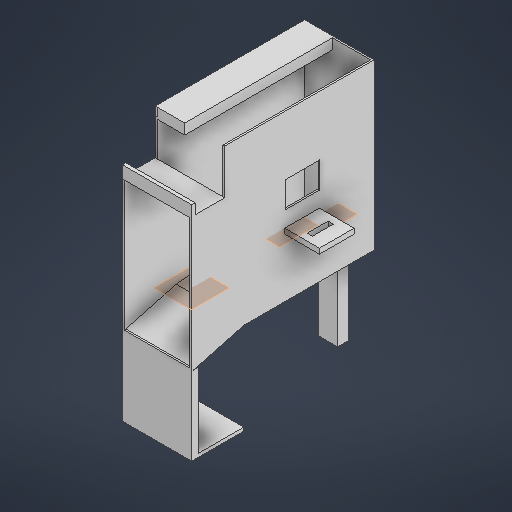
# Autodesk Inventor part: Na servo
Saved by Autodesk Inventor 2026.2 (Build 302298000, 298)
## iProperties
Created: 2026-03-13
Part Number: Na servo
Material: Všeobecné
Document SubType Name: Modeling
Designer: cerna
Density: 1 g/cm^3
Appearance: Výchozí
Author: cerna
Autodesk Inventor part; units mm, degrees
ref_plane "YZ Plane" through (0, 0, 0) normal (1, 0, 0) x (0, 1, 0)
ref_plane "XZ Plane" through (0, 0, 0) normal (0, 1, 0) x (-1, 0, 0)
ref_plane "XY Plane" through (0, 0, 0) normal (0, 0, 1) x (1, 0, 0)
sketch "Náčrt1" plane through (0, 0, 0) normal (0, 1, 0) x (-1, 0, 0)
  line L0 (20, 15) -> (-20, 15)
  line L1 (-20, 15) -> (-20, -15)
  line L2 (-20, -15) -> (20, -15)
  line L3 (20, -15) -> (20, 15)
  line L4 (0, -21) -> (0, 21) projected
  line L5 (-28, 0) -> (28, 0) projected
  point P0 (0, 0)
  dimension "d0" = 40
  dimension "d1" = 30
  constraints: 8 end point, 2 parallel, 1 horizontal, 1 perpendicular, 2 other
  measures "d0" distance of L2.end L1.end
  measures "d1" distance of L1.end L0.end
extrude "Vysunutí1" add sketch "Náčrt1" along normal blind 2
sketch "Náčrt2" plane through (0, 2, 0) normal (0, 1, 0) x (1, 0, 0)
  line L0 (-20, 15) -> (-20, -15) projected
  line L1 (-20, -15) -> (20, -15)
  line L2 (20, -15) -> (20, -14)
  line L3 (20, -14) -> (-20, -14)
  line L4 (-20, -14) -> (-20, -15)
  point P0 (0, 0)
  point P1 (-20, -14)
  dimension "d4" = 40
  dimension "d5" = 1
  constraints: 8 end point, 2 parallel, 1 horizontal, 1 perpendicular
  measures "d4" distance of L3.end L2.end
  measures "d5" distance of L2.end L1.end
extrude "Vysunutí2" add sketch "Náčrt2" along normal blind 44
sketch "Náčrt3" plane through (20, 0, 15) normal (1, 0, 0) x (0, 0, -1)
  line L0 (1, 2) -> (1, 46) projected
  line L1 (1, 45) -> (30.1328, 52.8061)
  line L2 (30.1328, 53.8061) -> (1, 46)
  line L3 (1, 46) -> (1, 45)
  line L4 (30.1328, 53.8061) -> (30.1328, 52.8061)
  line L5 (30, 0) -> (30, 2) projected
  line L6 (30.1328, 53.8061) -> (30.1328, 52.8061)
  line L7 (30.1328, 52.8061) -> (105.1328, 52.8061)
  line L8 (105.1328, 52.8061) -> (105.1328, 60.8061)
  line L9 (105.1328, 60.8061) -> (30.1328, 53.8061)
  point P0 (15, 0)
  point P1 (30.1328, 53.3061)
  dimension "d8" = 1
  dimension "d10" = 105
  dimension "d11" = 29.1328
  dimension "d59" = 75
  dimension "d60" = 8
  constraints: 16 end point, 2 perpendicular, 2 vertical, 1 collinear, 1 midpoint, 1 point on line
  measures "d8" distance of L1.start L0.end
  measures "d10" angle of L1 L0
  measures "d11" horizontal distance of L1.start L1.end
  measures "d59" distance of L1.end L7.end
  measures "d60" distance of L7.end L8.end
extrude "Vysunutí3" add sketch "Náčrt3" against normal blind 40
sketch "Náčrt5" plane through (20, 0, 15) normal (1, 0, 0) x (0, 0, -1)
  line L0 (53.6328, 89.524) -> (73.6328, 89.524)
  line L1 (73.6328, 89.524) -> (73.6328, 86.524)
  line L2 (73.6328, 86.524) -> (53.6328, 86.524)
  line L3 (53.6328, 86.524) -> (53.6328, 89.524)
  line L4 (0, 0) -> (30, 0) projected
  line L5 (30, 0) -> (30, 2) projected
  line L6 (1, 2) -> (30, 2) projected
  line L7 (1, 2) -> (1, 45) projected
  line L8 (1, 45) -> (30.1328, 52.8061) projected
  line L9 (30.1328, 53.8061) -> (1, 46) projected
  line L10 (0, 46) -> (1, 46) projected
  line L11 (0, 0) -> (0, 46) projected
  line L12 (67.1328, 89.524) -> (60.1328, 89.524) projected
  line L13 (63.6328, 89.524) -> (63.6328, 67.9806)
  line L14 (30.1328, 52.8061) -> (105.1328, 52.8061) projected
  line L15 (105.1328, 52.8061) -> (105.1328, 60.8061) projected
  line L16 (105.1328, 60.8061) -> (30.1328, 53.8061) projected
  point P0 (15, 0)
  dimension "d24" = 20
  dimension "d25" = 3
  constraints: 10 end point, 2 parallel, 1 collinear, 1 horizontal, 1 midpoint, 1 perpendicular, 1 vertical, 1 other
  measures "d24" distance between parallel lines of L1 L3
  measures "d25" distance between parallel lines of L0 L2
extrude "Vysunutí5" add sketch "Náčrt5" along normal blind 20 and the other way blind 3 contours L0 L13 L2 L3 | L0 L1 L2 L13
ref_plane "Pracovní rovina3" through (17, 89.524, -38.6328) normal (0, 1, 0) x (1, 0, 0)
sketch "Náčrt6" plane through (17, 89.524, -38.6328) normal (0, 1, 0) x (1, 0, 0)
  line L0 (0, 0) -> (0, 20) projected
  line L1 (0, 0) -> (23, 0) projected
  line L2 (23, 20) -> (23, 0) projected
  line L3 (0, 20) -> (23, 20) projected
  line L4 (3, 13.5) -> (3, 6.5) projected
  line L5 (0, 13.5) -> (3, 13.5) projected
  line L6 (3, 6.5) -> (0, 6.5) projected
  line L7 (12, 16) -> (15, 16)
  line L8 (15, 16) -> (15, 4)
  line L9 (15, 4) -> (12, 4)
  line L10 (12, 4) -> (12, 16)
  point P0 (-17, -38.6328)
  point P1 (12, 10)
  point P2 (0, 10)
  dimension "d30" = 12
  dimension "d31" = 3
  dimension "d32" = 12
  constraints: 8 end point, 2 midpoint, 2 parallel, 1 horizontal, 1 perpendicular
  measures "d30" distance of point (12, 10) point (0, 10)
  measures "d31" distance between parallel lines of L8 L10
  measures "d32" distance between parallel lines of L9 L7
extrude "Vysunutí6" cut sketch "Náčrt6" against normal blind 20 contours L7 L8 L9 L10
sketch "Náčrt7" plane through (20, 0, 15) normal (1, 0, 0) x (0, 0, -1)
  line L0 (60.1328, 55.5984) -> (30.1328, 53.8061) projected
  line L1 (30.1328, 53.8061) -> (1, 46) projected
  line L2 (0, 46) -> (1, 46) projected
  line L3 (0, 0) -> (0, 46) projected
  line L4 (0, 0) -> (30, 0) projected
  line L5 (30, 0) -> (30, 2) projected
  line L6 (1, 2) -> (30, 2) projected
  line L7 (1, 2) -> (1, 45) projected
  line L8 (1, 45) -> (30.1328, 52.8061) projected
  line L9 (0, 46) -> (0, 86.524)
  line L10 (0, 86.524) -> (97.0865, 86.524)
  line L11 (97.0865, 86.524) -> (97.0865, 57.8061)
  line L12 (30.1328, 53.8061) -> (0, 46)
  line L13 (30.1328, 52.8061) -> (105.1328, 52.8061) projected
  line L14 (105.1328, 52.8061) -> (105.1328, 60.8061) projected
  line L15 (105.1328, 60.8061) -> (30.1328, 53.8061) projected
  point P0 (15, 0)
  constraints: 8 end point, 2 perpendicular, 1 vertical
extrude "Vysunutí7" add sketch "Náčrt7" against normal blind 1 contours L1 L2 L12
sketch "Náčrt8" plane through (-20, 0, -15) normal (-1, 0, 0) x (0, 0, 1)
  line L0 (0, 0) -> (30, 0) projected
  line L1 (30, 0) -> (30, 46) projected
  line L2 (29, 46) -> (30, 46) projected
  line L3 (29, 46) -> (-0.1328, 53.8061) projected
  line L4 (-0.1328, 52.8061) -> (29, 45) projected
  line L5 (29, 2) -> (29, 45) projected
  line L6 (0, 2) -> (29, 2) projected
  line L7 (0, 0) -> (0, 2) projected
  line L8 (-67.0865, 57.8061) -> (-67.0865, 86.524) projected
  line L9 (-67.0865, 57.8061) -> (-67.0865, 60.0551)
  line L10 (-23.6328, 86.524) -> (30, 86.524) projected
  line L11 (29, 86.524) -> (30, 86.524)
  line L12 (30, 52.0059) -> (30, 50.9937)
  line L13 (29, 46) -> (-0.1328, 53.8061) projected
  line L14 (-0.1328, 53.8061) -> (-67.0865, 57.8061) projected
  line L15 (-0.1328, 53.8061) -> (-67.0865, 57.8061)
  line L16 (-67.0865, 57.8061) -> (-67.0865, 60.0551)
  line L17 (-0.1328, 53.8061) -> (-75.1328, 60.8061) projected
  line L18 (-75.1328, 60.8061) -> (-75.1328, 52.8061) projected
  line L19 (-75.1328, 52.8061) -> (-0.1328, 52.8061) projected
  line L20 (-67.0865, 60.0551) -> (-75.1328, 60.8061)
  line L21 (-75.1328, 73.9023) -> (-75.1328, 72.9023)
  line L22 (30, 46) -> (-75.1328, 46)
  line L23 (-75.1328, 46) -> (-75.1328, 143)
  line L24 (-75.1328, 143) -> (30, 143)
  line L25 (30, 143) -> (30, 46)
  point P0 (15, 0)
  point P1 (29, 86.524)
  dimension "d76" = 97
  constraints: 22 end point, 6 point on line, 4 collinear, 3 parallel, 1 horizontal, 1 perpendicular, 1 vertical
  measures "d76" distance of L22.end L23.end
extrude "Vysunutí8" add sketch "Náčrt8" against normal blind 1 contours L2 L3 L17 L23 L21 L24 L25 L12 | L14 L8 L17
ref_plane "Pracovní rovina1" through (20, 86.524, -58.6328) normal (0, 1, 0) x (1, 0, 0)
ref_plane "Pracovní rovina2" through (20, 86.524, 15) normal (0, 1, 0) x (1, 0, 0)
sketch "Náčrt14" plane through (20, 0, 15) normal (1, 0, 0) x (0, 0, -1)
  line L0 (0, 46) -> (0, 141.524) projected
  line L1 (0, 120.8494) -> (17, 120.8494)
  line L2 (17, 120.8494) -> (17, 155.8494)
  line L3 (17, 155.8494) -> (0, 155.8494)
  line L4 (0, 155.8494) -> (0, 120.8494)
  point P0 (15, 0)
  dimension "d50" = 17
  dimension "d51" = 35
  constraints: 8 end point, 2 parallel, 1 horizontal, 1 perpendicular, 1 point on line
  measures "d50" distance of L3.end L2.end
  measures "d51" distance of L2.end L1.end
extrude "Vysunutí14" cut sketch "Náčrt14" against normal blind 100
sketch "Náčrt15" plane through (20, 52.8061, -90.1328) normal (0, 0, -1) x (-1, 0, 0)
  line L0 (0, 0) -> (0, 8) projected
  line L1 (0, 0) -> (40, 0) projected
  line L2 (0, 8) -> (39, 8) projected
  line L3 (0, 0) -> (40.66, 0)
  line L4 (40.66, 0) -> (40.66, 90)
  line L5 (40.66, 90) -> (0, 90)
  line L6 (0, 90) -> (0, 0)
  line L7 (40, 90.1939) -> (40, 0) projected
  line L8 (40, 90.1939) -> (39, 90.1939) projected
  line L9 (39, 8) -> (39, 90.1939) projected
  point P0 (20, -52.8061)
  point P1 (40, 0)
  point P2 (40, 90)
  point P3 (39, 90)
  dimension "d62" = 90
  constraints: 8 end point, 2 parallel, 1 horizontal, 1 perpendicular
  measures "d62" distance of L4.end L3.end
extrude "Vysunutí15" add sketch "Náčrt15" against normal blind 1 contours L6 L5 L9 L2 | L7 L5 L4 L3
sketch "Náčrt16" plane through (20, 0, 15) normal (1, 0, 0) x (0, 0, -1)
  line L0 (105.1328, 60.8061) -> (30.1328, 53.8061) projected
  line L1 (30.1328, 53.8061) -> (0, 46) projected
  line L2 (0, 0) -> (0, 46) projected
  line L3 (0, 0) -> (30, 0) projected
  line L4 (30, 0) -> (30, 2) projected
  line L5 (1, 2) -> (30, 2) projected
  line L6 (1, 2) -> (1, 45) projected
  line L7 (1, 45) -> (30.1328, 52.8061) projected
  line L8 (30.1328, 52.8061) -> (105.1328, 52.8061) projected
  line L9 (105.1328, 52.8061) -> (105.1328, 60.8061) projected
  line L10 (105.1328, 142.8061) -> (105.1328, 60.8061) projected
  line L11 (0, 46) -> (105.1328, 46)
  line L12 (105.1328, 46) -> (105.1328, 142.8061)
  line L13 (105.1328, 142.8061) -> (0, 142.8061)
  line L14 (0, 142.8061) -> (0, 46)
  line L15 (0, 46) -> (30.1328, 53.8061)
  line L16 (60.1328, 56.6061) -> (30.1328, 53.8061) projected
  line L17 (30.1328, 53.8061) -> (60.1328, 56.6061)
  line L18 (60.1328, 56.6061) -> (105.1328, 60.8061)
  line L19 (60.1328, 56.6061) -> (105.1328, 60.8061)
  point P0 (15, 0)
  constraints: 16 end point, 4 equal length, 1 horizontal, 1 perpendicular, 1 point on line
extrude "Vysunutí16" add sketch "Náčrt16" against normal blind 1 contours L0 L1 L14 L13 L10
sketch "Náčrt17" plane through (20, 0, 15) normal (1, 0, 0) x (0, 0, -1)
  line L0 (54.254, 98.524) -> (73.8811, 98.524)
  line L1 (73.8811, 98.524) -> (73.8811, 113.524)
  line L2 (73.8811, 113.524) -> (54.254, 113.524)
  line L3 (54.254, 113.524) -> (54.254, 98.524)
  line L4 (53.6328, 86.524) -> (73.6328, 86.524) projected
  line L5 (53.6328, 86.524) -> (73.6328, 86.524) projected
  line L6 (73.6328, 86.524) -> (73.6328, 89.524) projected
  line L7 (73.6328, 89.524) -> (53.6328, 89.524) projected
  line L8 (53.6328, 89.524) -> (53.6328, 86.524) projected
  point P0 (15, 0)
  dimension "d67" = 9
  dimension "d68" = 15
  constraints: 8 end point, 2 parallel, 1 horizontal, 1 perpendicular
  measures "d67" distance between parallel lines of L0 L7
  measures "d68" distance between parallel lines of L2 L0
extrude "Vysunutí17" cut sketch "Náčrt17" against normal blind 1 contours L3 L2 L1 L0
sketch "Náčrt18" plane through (20, 0, 15) normal (1, 0, 0) x (0, 0, -1)
  line L0 (54.254, 113.524) -> (73.8811, 113.524) projected
  line L1 (73.8811, 113.524) -> (73.8811, 98.524) projected
  line L2 (73.8811, 98.524) -> (54.254, 98.524) projected
  line L3 (54.254, 98.524) -> (54.254, 113.524) projected
  line L4 (53.6328, 86.524) -> (73.6328, 86.524) projected
  line L5 (53.6328, 89.524) -> (53.6328, 86.524) projected
  line L6 (73.6328, 89.524) -> (53.6328, 89.524) projected
  line L7 (73.6328, 86.524) -> (73.6328, 89.524) projected
  line L8 (105.1328, 52.8061) -> (105.1328, 142.8061) projected
  line L9 (105.1328, 142.8061) -> (0, 142.8061) projected
  line L10 (0, 0) -> (0, 142.8061) projected
  line L11 (0, 0) -> (30, 0) projected
  line L12 (30, 0) -> (30, 2) projected
  line L13 (1, 2) -> (30, 2) projected
  line L14 (1, 2) -> (1, 45) projected
  line L15 (1, 45) -> (30.1328, 52.8061) projected
  line L16 (30.1328, 52.8061) -> (105.1328, 52.8061) projected
  line L17 (105.1328, 142.8061) -> (0, 142.8061) projected
  line L18 (0, 122) -> (19, 122)
  line L19 (19, 122) -> (19, 142.8061)
  line L20 (19, 142.8061) -> (0, 142.8061)
  line L21 (0, 142.8061) -> (0, 122)
  point P0 (15, 0)
  dimension "d71" = 77
  dimension "d72" = 19
  constraints: 8 end point, 2 parallel, 2 point on line, 1 horizontal, 1 perpendicular
  measures "d71" distance from line of L18 L14.end
  measures "d72" distance of L18.start L18.end
extrude "Vysunutí18" cut sketch "Náčrt18" against normal blind 60 contours L19 L18 L10 L9
sketch "Náčrt19" plane through (20, 122, 15) normal (0, 1, 0) x (1, 0, 0)
  line L0 (0, 19) -> (0, 0) projected
  line L1 (-40, 17) -> (-40, 19) projected
  line L2 (0, 19) -> (-40, 19)
  line L3 (-40, 19) -> (-40, 0)
  line L4 (-40, 0) -> (0, 0)
  line L5 (0, 0) -> (0, 19)
  point P0 (-20, 15)
  constraints: 8 end point, 2 parallel, 1 horizontal, 1 perpendicular
extrude "Vysunutí19" add sketch "Náčrt19" against normal blind 1
sketch "Náčrt20" plane through (17, 89.524, -38.6328) normal (0, 1, 0) x (1, 0, 0)
  line L0 (0, 20) -> (2, 20) projected
  line L1 (2, 20) -> (0, 20)
  line L2 (0, 20) -> (0, 0)
  line L3 (0, 0) -> (2, 0)
  line L4 (2, 0) -> (2, 20)
  point P0 (-17, -38.6328)
  constraints: 8 end point, 2 parallel, 1 horizontal, 1 perpendicular
extrude "Vysunutí20" cut sketch "Náčrt20" against normal blind 10
sketch "Náčrt21" plane through (20, 52.8061, -89.1328) normal (0, 0, 1) x (1, 0, 0)
  line L0 (-40.66, 90) -> (-40.66, 0) projected
  line L1 (-1, 90) -> (-40.66, 90) projected
  line L2 (-1, 8) -> (-1, 90) projected
  line L3 (-1, 90) -> (-39, 90) projected
  line L4 (-40.66, 90) -> (-40.66, 0) projected
  line L5 (-40.66, 0) -> (-40, 0) projected
  line L6 (-40, 90) -> (-40, 0) projected
  line L7 (-39, 8) -> (-39, 90) projected
  line L8 (-39, 8) -> (-1, 8) projected
  line L9 (-40, 90) -> (-40.66, 90)
  line L10 (-40.66, 90) -> (-40.66, 0)
  line L11 (-40.66, 0) -> (-40, 0)
  line L12 (-40, 0) -> (-40, 90)
  line L13 (-40, 90) -> (-40.66, 90) projected
  point P0 (-20, -52.8061)
  constraints: 8 end point, 2 parallel, 1 horizontal, 1 perpendicular, 1 point on line
extrude "Vysunutí21" cut sketch "Náčrt21" against normal blind 10 contours L1 L6 L5 L0
sketch "Náčrt22" plane through (-19, 142.8061, -90.1328) normal (0, 1, 0) x (1, 0, 0)
  line L0 (38, -1) -> (0, -1) projected
  line L1 (-1, -88.1328) -> (-1, 0) projected
  line L2 (-1, -88.1328) -> (0, -88.1328) projected
  line L3 (0, 0) -> (0, -88.1328) projected
  line L4 (-1, 0) -> (0, 0) projected
  line L5 (-1, -88.1328) -> (-1, 0) projected
  line L6 (0, 0) -> (39, 0) projected
  line L7 (16, 0) -> (-1, 0)
  line L8 (-1, 0) -> (-1, -86.1328)
  line L9 (-1, -86.1328) -> (16, -86.1328)
  line L10 (16, -86.1328) -> (16, 0)
  line L11 (38, -86.1328) -> (38, -1) projected
  line L12 (-1, -105.1328) -> (-1, -88.1328) projected
  line L13 (38, -105.1328) -> (-1, -105.1328) projected
  line L14 (0, -86.1328) -> (38, -86.1328) projected
  line L15 (38, -105.1328) -> (38, -86.1328) projected
  line L16 (0, -88.1328) -> (-1, -88.1328) projected
  line L17 (0, -86.1328) -> (0, -88.1328) projected
  point P0 (19, -90.1328)
  point P1 (16, -1)
  dimension "d83" = 22
  constraints: 8 end point, 2 parallel, 2 point on line, 1 collinear, 1 horizontal, 1 perpendicular
  measures "d83" distance between parallel lines of L10 L11
extrude "Vysunutí22" add sketch "Náčrt22" against normal blind 1 contours L10 L9 L3 L0
sketch "Náčrt23" plane through (-20, 143, -2) normal (0, 1, 0) x (1, 0, 0)
  line L0 (1, 88.1328) -> (1, 0) projected
  line L1 (0, 13) -> (0, -17) projected
  line L2 (1, 88.1328) -> (0, 88.1328)
  line L3 (0, 88.1328) -> (0, -0.0197)
  line L4 (0, -0.0197) -> (1, -0.0197)
  line L5 (1, -0.0197) -> (1, 88.1328)
  point P0 (20, -2)
  point P1 (1, 0)
  constraints: 8 end point, 2 parallel, 1 horizontal, 1 perpendicular, 1 point on line
extrude "Vysunutí23" cut sketch "Náčrt23" against normal blind 0.195
sketch "Náčrt24" plane through (-20, 0, 15) normal (0, 0, 1) x (1, 0, 0)
  line L0 (40, 122) -> (0, 122) projected
  line L1 (39, 121) -> (0, 121) projected
  line L2 (40, 142.8061) -> (40, 122) projected
  line L3 (0, 121) -> (40, 121)
  line L4 (40, 121) -> (40, 128)
  line L5 (40, 128) -> (0, 128)
  line L6 (0, 128) -> (0, 121)
  point P0 (20, 0)
  dimension "d88" = 7
  constraints: 8 end point, 2 parallel, 1 horizontal, 1 perpendicular, 1 point on line
  measures "d88" distance of L4.end L3.end
extrude "Vysunutí24" add sketch "Náčrt24" against normal blind 2 contours L0 L6 L5 L2
sketch "Náčrt25" plane through (20, 52.8061, -90.1328) normal (0, -1, 0) x (1, 0, 0)
  line L0 (-1, 0) -> (-39, 0) projected
  line L1 (-15, 0) -> (-26, 0)
  line L2 (-26, 0) -> (-26, 6)
  line L3 (-26, 6) -> (-15, 6)
  line L4 (-15, 6) -> (-15, 0)
  point P0 (-20, 90.1328)
  point P1 (-20.5, 6)
  point P2 (-26, 0)
  dimension "d91" = 11
  dimension "d92" = 6
  dimension "d93" = 19.5
  constraints: 8 end point, 2 parallel, 1 horizontal, 1 midpoint, 1 perpendicular, 1 point on line
  measures "d91" distance of L2.end L3.end
  measures "d92" distance of L1.end L2.end
  measures "d93" horizontal distance of L0.start point (-20.5, 6)
extrude "Vysunutí25" add sketch "Náčrt25" along normal blind 52.806
sketch "Náčrt26" plane through (20, 2, 14) normal (0, 0, -1) x (-1, 0, 0)
  line L0 (40, 43) -> (0, 43) projected
  line L1 (0, 0) -> (0, 43) projected
  line L2 (40, 0) -> (0, 0) projected
  line L3 (40, 0) -> (40, 43) projected
  line L4 (0, 43) -> (40, 43)
  line L5 (40, 43) -> (40, 0)
  line L6 (40, 0) -> (0, 0)
  line L7 (0, 0) -> (0, 43)
  point P0 (20, -2)
  constraints: 8 end point, 2 parallel, 1 horizontal, 1 perpendicular
extrude "Vysunutí26" add sketch "Náčrt26" along normal blind 3
sketch "Náčrt27" plane through (20, 142.8061, -4) normal (0, 1, 0) x (1, 0, 0)
  line L0 (-40, 11) -> (-40, -15) projected
  line L1 (-1, 86.1328) -> (-39, 86.1328) projected
  line L2 (-40, 0.079) -> (-22.8867, 0.079)
  line L3 (-22.8867, 0.079) -> (-22.8867, 86.1328)
  line L4 (-22.8867, 86.1328) -> (-40, 86.1328)
  line L5 (-40, 86.1328) -> (-40, 0.079)
  line L6 (-1, 0) -> (0, 0) projected
  line L7 (0, 86.1328) -> (0, 0) projected
  line L8 (-39, 86.1328) -> (0, 86.1328) projected
  line L9 (-39, 0) -> (-39, 86.1328) projected
  line L10 (-39, 0) -> (-23, 0) projected
  line L11 (-23, 0) -> (-23, 85.1328) projected
  line L12 (-1, 85.1328) -> (-23, 85.1328) projected
  line L13 (-1, 0) -> (-1, 85.1328) projected
  line L14 (-1, 0) -> (0, 0)
  line L15 (0, 0) -> (0, 86.1328)
  line L16 (0, 86.1328) -> (-1, 86.1328)
  line L17 (-1, 86.1328) -> (-1, 0)
  line L18 (-26, 86.1328) -> (-40, 86.1328) projected
  line L19 (-40, 86.1328) -> (0, 86.1328)
  line L20 (0, 86.1328) -> (0, 85.1328)
  line L21 (0, 85.1328) -> (-40, 85.1328)
  line L22 (-40, 85.1328) -> (-40, 86.1328)
  line L23 (-40, 0.079) -> (-23, 0.079)
  line L24 (-23, 0.079) -> (-23, 85.1328)
  line L25 (-23, 85.1328) -> (-40, 85.1328)
  line L26 (-40, 85.1328) -> (-40, 0.079)
  point P0 (-20, -4)
  point P1 (-39, 0.079)
  constraints: 32 end point, 8 parallel, 4 horizontal, 4 perpendicular, 4 point on line
extrude "Vysunutí27" add sketch "Náčrt27" along normal blind 5 contours L5 L21 L9 L2 L0 | L5 L4 L9 L21 | L9 L21 L11 L2 | L2 L11 L10 L9 | L9 L1 L3 L12 L21 | L3 L1 L17 L12 | L21 L7 L6 L13 | L17 L8 L7 L21
